Autodesk Inventor part; units mm, degrees
(part 2 of 3)
  line L955 (9.481, 12.2224) -> (9.3887, 12.173)
  line L956 (9.3887, 12.173) -> (9.2008, 12.0779)
  line L957 (9.2008, 12.0779) -> (8.8135, 11.9014)
  line L958 (8.8135, 11.9014) -> (8.4127, 11.7415)
  line L959 (8.4127, 11.7415) -> (7.9999, 11.5967)
  line L960 (7.9999, 11.5967) -> (7.5762, 11.4663)
  line L961 (7.5762, 11.4663) -> (7.1423, 11.3497)
  line L962 (7.1423, 11.3497) -> (6.777, 11.8009)
  line L963 (6.777, 11.8009) -> (6.9813, 12.201)
  line L964 (6.9813, 12.201) -> (7.1969, 12.5884)
  line L965 (7.1969, 12.5884) -> (7.4243, 12.9621)
  line L966 (7.4243, 12.9621) -> (7.6641, 13.3208)
  line L967 (7.6641, 13.3208) -> (7.9172, 13.663)
  line L968 (7.9172, 13.663) -> (8.0493, 13.827)
  line L969 (8.0493, 13.827) -> (8.1169, 13.907)
  line L970 (8.1169, 13.907) -> (8.1855, 13.9856)
  line L971 (8.1855, 13.9856) -> (7.7098, 14.6404)
  line L972 (7.7098, 14.6404) -> (7.6138, 14.5994)
  line L973 (7.6138, 14.5994) -> (7.5168, 14.5599)
  line L974 (7.5168, 14.5599) -> (7.32, 14.4849)
  line L975 (7.32, 14.4849) -> (6.9164, 14.3499)
  line L976 (6.9164, 14.3499) -> (6.5011, 14.2327)
  line L977 (6.5011, 14.2327) -> (6.0755, 14.1319)
  line L978 (6.0755, 14.1319) -> (5.6404, 14.0465)
  line L979 (5.6404, 14.0465) -> (5.1967, 13.9759)
  line L980 (5.1967, 13.9759) -> (4.8805, 14.4628)
  line L981 (4.8805, 14.4628) -> (5.1255, 14.8394)
  line L982 (5.1255, 14.8394) -> (5.3805, 15.2021)
  line L983 (5.3805, 15.2021) -> (5.6457, 15.55)
  line L984 (5.6457, 15.55) -> (5.9217, 15.8817)
  line L985 (5.9217, 15.8817) -> (6.2092, 16.1955)
  line L986 (6.2092, 16.1955) -> (6.3577, 16.3448)
  line L987 (6.3577, 16.3448) -> (6.4333, 16.4173)
  line L988 (6.4333, 16.4173) -> (6.5097, 16.4883)
  line L989 (6.5097, 16.4883) -> (6.1051, 17.1892)
  line L990 (6.1051, 17.1892) -> (6.0053, 17.1585)
  line L991 (6.0053, 17.1585) -> (5.9047, 17.1293)
  line L992 (5.9047, 17.1293) -> (5.7012, 17.0754)
  line L993 (5.7012, 17.0754) -> (5.2857, 16.9833)
  line L994 (5.2857, 16.9833) -> (4.8604, 16.9101)
  line L995 (4.8604, 16.9101) -> (4.4265, 16.8544)
  line L996 (4.4265, 16.8544) -> (3.9849, 16.8149)
  line L997 (3.9849, 16.8149) -> (3.5363, 16.7911)
  line L998 (3.5363, 16.7911) -> (3.2727, 17.3084)
  line L999 (3.2727, 17.3084) -> (3.5558, 17.6573)
  line L1000 (3.5558, 17.6573) -> (3.8472, 17.9913)
  line L1001 (3.8472, 17.9913) -> (4.1474, 18.3096)
  line L1002 (4.1474, 18.3096) -> (4.4565, 18.6106)
  line L1003 (4.4565, 18.6106) -> (4.7752, 18.8927)
  line L1004 (4.7752, 18.8927) -> (4.9385, 19.0256)
  line L1005 (4.9385, 19.0256) -> (5.0212, 19.0899)
  line L1006 (5.0212, 19.0899) -> (5.1047, 19.1525)
  line L1007 (5.1047, 19.1525) -> (4.7756, 19.8919)
  line L1008 (4.7756, 19.8919) -> (4.6731, 19.8717)
  line L1009 (4.6731, 19.8717) -> (4.5701, 19.8532)
  line L1010 (4.5701, 19.8532) -> (4.362, 19.8208)
  line L1011 (4.362, 19.8208) -> (3.9391, 19.7727)
  line L1012 (3.9391, 19.7727) -> (3.5085, 19.7444)
  line L1013 (3.5085, 19.7444) -> (3.0712, 19.7343)
  line L1014 (3.0712, 19.7343) -> (2.6279, 19.7412)
  line L1015 (2.6279, 19.7412) -> (2.1792, 19.7644)
  line L1016 (2.1792, 19.7644) -> (1.9712, 20.3064)
  line L1017 (1.9712, 20.3064) -> (2.2891, 20.6238)
  line L1018 (2.2891, 20.6238) -> (2.6139, 20.9256)
  line L1019 (2.6139, 20.9256) -> (2.9457, 21.2107)
  line L1020 (2.9457, 21.2107) -> (3.2846, 21.4778)
  line L1021 (3.2846, 21.4778) -> (3.631, 21.725)
  line L1022 (3.631, 21.725) -> (3.8074, 21.8401)
  line L1023 (3.8074, 21.8401) -> (3.8963, 21.8954)
  line L1024 (3.8963, 21.8954) -> (3.9859, 21.949)
  line L1025 (3.9859, 21.949) -> (3.7358, 22.7186)
  line L1026 (3.7358, 22.7186) -> (3.6319, 22.7093)
  line L1027 (3.6319, 22.7093) -> (3.5274, 22.7017)
  line L1028 (3.5274, 22.7017) -> (3.3171, 22.6913)
  line L1029 (3.3171, 22.6913) -> (2.8915, 22.6876)
  line L1030 (2.8915, 22.6876) -> (2.4603, 22.7045)
  line L1031 (2.4603, 22.7045) -> (2.0243, 22.7401)
  line L1032 (2.0243, 22.7401) -> (1.5842, 22.7933)
  line L1033 (1.5842, 22.7933) -> (1.1404, 22.8633)
  line L1034 (1.1404, 22.8633) -> (0.9901, 23.4241)
  line L1035 (0.9901, 23.4241) -> (1.3395, 23.7065)
  line L1036 (1.3395, 23.7065) -> (1.6941, 23.9727)
  line L1037 (1.6941, 23.9727) -> (2.0538, 24.2216)
  line L1038 (2.0538, 24.2216) -> (2.4188, 24.4518)
  line L1039 (2.4188, 24.4518) -> (2.7892, 24.6613)
  line L1040 (2.7892, 24.6613) -> (2.9766, 24.7575)
  line L1041 (2.9766, 24.7575) -> (3.0708, 24.8031)
  line L1042 (3.0708, 24.8031) -> (3.1655, 24.847)
  line L1043 (3.1655, 24.847) -> (2.9973, 25.6386)
  line L1044 (2.9973, 25.6386) -> (2.8929, 25.6402)
  line L1045 (2.8929, 25.6402) -> (2.7882, 25.6436)
  line L1046 (2.7882, 25.6436) -> (2.5779, 25.6552)
  line L1047 (2.5779, 25.6552) -> (2.1543, 25.696)
  line L1048 (2.1543, 25.696) -> (1.7273, 25.7578)
  line L1049 (1.7273, 25.7578) -> (1.2974, 25.8389)
  line L1050 (1.2974, 25.8389) -> (0.8652, 25.9378)
  line L1051 (0.8652, 25.9378) -> (0.4312, 26.0538)
  line L1052 (0.4312, 26.0538) -> (0.3404, 26.6272)
  line L1053 (0.3404, 26.6272) -> (0.7173, 26.8716)
  line L1054 (0.7173, 26.8716) -> (1.0978, 27.0992)
  line L1055 (1.0978, 27.0992) -> (1.4816, 27.3091)
  line L1056 (1.4816, 27.3091) -> (1.8686, 27.4999)
  line L1057 (1.8686, 27.4999) -> (2.2589, 27.6697)
  line L1058 (2.2589, 27.6697) -> (2.4553, 27.7456)
  line L1059 (2.4553, 27.7456) -> (2.5538, 27.7812)
  line L1060 (2.5538, 27.7812) -> (2.6526, 27.8149)
  line L1061 (2.6526, 27.8149) -> (2.568, 28.6198)
  line L1062 (2.568, 28.6198) -> (2.4644, 28.6323)
  line L1063 (2.4644, 28.6323) -> (2.3606, 28.6466)
  line L1064 (2.3606, 28.6466) -> (2.1527, 28.6801)
  line L1065 (2.1527, 28.6801) -> (1.7356, 28.765)
  line L1066 (1.7356, 28.765) -> (1.3174, 28.8711)
  line L1067 (1.3174, 28.8711) -> (0.8983, 28.9967)
  line L1068 (0.8983, 28.9967) -> (0.4789, 29.1403)
  line L1069 (0.4789, 29.1403) -> (0.0593, 29.3009)
  line L1070 (0.0593, 29.3009) -> (0.029, 29.8807)
  line L1071 (0.029, 29.8807) -> (0.4294, 30.0843)
  line L1072 (0.4294, 30.0843) -> (0.8316, 30.2709)
  line L1073 (0.8316, 30.2709) -> (1.2352, 30.4396)
  line L1074 (1.2352, 30.4396) -> (1.64, 30.5889)
  line L1075 (1.64, 30.5889) -> (2.0459, 30.7169)
  line L1076 (2.0459, 30.7169) -> (2.2492, 30.772)
  line L1077 (2.2492, 30.772) -> (2.3509, 30.797)
  line L1078 (2.3509, 30.797) -> (2.4527, 30.8203)
  line L1079 (2.4527, 30.8203) -> (2.4527, 31.6296)
  circle A0 centre (31.2249, 31.2249) radius 0.5
  line L1080 (62.4057, 32.859) -> (0.0441, 29.5908) construction
derived "Base_part.ipt"
sketch "Sketch7" plane through (0, 0, 0) normal (0, 1, 0) x (-1, 0, 0)
  line L0 (0.8173, 31.2129) -> (-0.8173, -31.2129) construction
  arc A0 (27.3185, 5) -> (4, 27.4827) centre (0, 0) ccw
  line L1 (5, 14.1421) -> (5, 27.3185)
  line L2 (4, 14.4568) -> (4, 27.4827)
  arc A1 (5, 27.3185) -> (4, 27.4827) centre (0, 0) ccw
  arc A2 (0.727, 27.7627) -> (27.4827, 4) centre (0, 0) ccw
  arc A3 (14.9718, 8.0526) -> (8.0526, 14.9718) centre (0, 0) ccw
  line L3 (16.7332, 7) -> (22.0027, 7)
  line L4 (7, 16.7332) -> (7, 22.0027)
  arc A4 (23.8539, 9.7572) -> (9.7572, 23.8539) centre (0, 0) ccw
  arc A5 (22.0027, 7) -> (23.8539, 9.7572) centre (22.0027, 9) ccw
  arc A6 (14.9718, 8.0526) -> (16.7332, 7) centre (16.7332, 9) ccw
  arc A7 (7, 16.7332) -> (8.0526, 14.9718) centre (9, 16.7332) ccw
  arc A8 (9.7572, 23.8539) -> (7, 22.0027) centre (9, 22.0027) ccw
  line L5 (0, 0) -> (0, -11.3594) construction
  arc A9 (14.1421, 5) -> (5, 14.1421) centre (0, 0) ccw
  line L6 (14.1421, 5) -> (27.3185, 5)
  line L7 (0, 0) -> (-23.3168, 0) construction
  line L8 (27.4827, 4) -> (14.4568, 4)
  arc A10 (14.4568, 4) -> (14.1421, 5) centre (0, 0) ccw
  arc A11 (4, 14.4568) -> (14.4568, 4) centre (0, 0) ccw
  arc A12 (5, 14.1421) -> (4, 14.4568) centre (0, 0) ccw
  arc A13 (27.3185, 5) -> (5, 27.3185) centre (0, 0) ccw
  arc A14 (27.4827, 4) -> (27.3185, 5) centre (0, 0) ccw
  arc A15 (4, 27.4827) -> (-14.6783, 23.5764) centre (0, 0) ccw
  arc A16 (-4, 14.4568) -> (-5, 14.1421) centre (0, 0) ccw
  line L9 (-4, 27.4827) -> (-4, 14.4568)
  arc A17 (-4, 27.4827) -> (-5, 27.3185) centre (0, 0) ccw
  line L10 (-5, 14.1421) -> (-5, 27.3185)
  arc A18 (-14.1421, 5) -> (-14.4568, 4) centre (0, 0) ccw
  line L11 (-14.1421, 5) -> (-27.3184, 5)
  line L12 (-14.4568, 4) -> (-27.4827, 4)
  arc A19 (-27.3184, 5) -> (-27.4827, 4) centre (0, 0) ccw
  arc A20 (-23.8538, 9.7572) -> (-22.0027, 7) centre (-22.0027, 9) ccw
  arc A21 (-9.7572, 23.8539) -> (-23.8538, 9.7572) centre (0, 0) ccw
  arc A22 (-8.0526, 14.9718) -> (-14.9718, 8.0526) centre (0, 0) ccw
  arc A23 (-16.7332, 7) -> (-14.9718, 8.0526) centre (-16.7332, 9) ccw
  line L13 (-16.7332, 7) -> (-22.0027, 7)
  arc A24 (-8.0526, 14.9718) -> (-7, 16.7332) centre (-9, 16.7332) ccw
  arc A25 (-7, 22.0027) -> (-9.7572, 23.8539) centre (-9, 22.0027) ccw
  line L14 (-7, 16.7332) -> (-7, 22.0027)
  arc A26 (-14.4568, -4) -> (-14.1421, -5) centre (0, 0) ccw
  line L15 (-27.4827, -4) -> (-14.4568, -4)
  arc A27 (-27.4827, -4) -> (-27.3184, -5) centre (0, 0) ccw
  line L16 (-14.1421, -5) -> (-27.3184, -5)
  arc A28 (-5, -14.1421) -> (-4, -14.4568) centre (0, 0) ccw
  line L17 (-5, -14.1421) -> (-5, -27.3184)
  line L18 (-4, -14.4568) -> (-4, -27.4827)
  arc A29 (-5, -27.3184) -> (-4, -27.4827) centre (0, 0) ccw
  arc A30 (-9.7572, -23.8538) -> (-7, -22.0027) centre (-9, -22.0027) ccw
  arc A31 (-23.8538, -9.7572) -> (-9.7572, -23.8538) centre (0, 0) ccw
  arc A32 (-14.9718, -8.0526) -> (-8.0526, -14.9718) centre (0, 0) ccw
  arc A33 (-7, -16.7332) -> (-8.0526, -14.9718) centre (-9, -16.7332) ccw
  line L19 (-7, -16.7332) -> (-7, -22.0027)
  arc A34 (-14.9718, -8.0526) -> (-16.7332, -7) centre (-16.7332, -9) ccw
  arc A35 (-22.0027, -7) -> (-23.8538, -9.7572) centre (-22.0027, -9) ccw
  line L20 (-16.7332, -7) -> (-22.0027, -7)
  arc A36 (4, -14.4568) -> (5, -14.1421) centre (0, 0) ccw
  line L21 (4, -27.4827) -> (4, -14.4568)
  arc A37 (4, -27.4827) -> (5, -27.3184) centre (0, 0) ccw
  line L22 (5, -14.1421) -> (5, -27.3184)
  arc A38 (14.1421, -5) -> (14.4568, -4) centre (0, 0) ccw
  line L23 (14.1421, -5) -> (27.3185, -5)
  line L24 (14.4568, -4) -> (27.4827, -4)
  arc A39 (27.3185, -5) -> (27.4827, -4) centre (0, 0) ccw
  arc A40 (23.8539, -9.7572) -> (22.0027, -7) centre (22.0027, -9) ccw
  arc A41 (9.7572, -23.8538) -> (23.8539, -9.7572) centre (0, 0) ccw
  arc A42 (8.0526, -14.9718) -> (14.9718, -8.0526) centre (0, 0) ccw
  arc A43 (16.7332, -7) -> (14.9718, -8.0526) centre (16.7332, -9) ccw
  line L25 (16.7332, -7) -> (22.0027, -7)
  arc A44 (8.0526, -14.9718) -> (7, -16.7332) centre (9, -16.7332) ccw
  arc A45 (7, -22.0027) -> (9.7572, -23.8538) centre (9, -22.0027) ccw
  line L26 (7, -16.7332) -> (7, -22.0027)
  line L27 (-28.6518, 2.6609) -> (-28.7514, 2.692)
  line L28 (-28.7514, 2.692) -> (-28.8508, 2.725)
  line L29 (-28.8508, 2.725) -> (-29.0492, 2.7958)
  line L30 (-29.0492, 2.7958) -> (-29.4438, 2.9552)
  line L31 (-29.4438, 2.9552) -> (-29.8357, 3.1359)
  line L32 (-29.8357, 3.1359) -> (-30.2248, 3.3356)
  line L33 (-30.2248, 3.3356) -> (-30.6111, 3.5533)
  line L34 (-30.6111, 3.5533) -> (-30.9943, 3.7877)
  line L35 (-30.9943, 3.7877) -> (-30.9185, 4.3633)
  line L36 (-30.9185, 4.3633) -> (-30.4877, 4.4905)
  line L37 (-30.4877, 4.4905) -> (-30.0582, 4.6008)
  line L38 (-30.0582, 4.6008) -> (-29.6306, 4.693)
  line L39 (-29.6306, 4.693) -> (-29.2054, 4.7661)
  line L40 (-29.2054, 4.7661) -> (-28.7829, 4.8179)
  line L41 (-28.7829, 4.8179) -> (-28.573, 4.835)
  line L42 (-28.573, 4.835) -> (-28.4685, 4.8411)
  line L43 (-28.4685, 4.8411) -> (-28.3642, 4.8454)
  line L44 (-28.3642, 4.8454) -> (-28.2167, 5.6412)
  line L45 (-28.2167, 5.6412) -> (-28.3125, 5.6826)
  line L46 (-28.3125, 5.6826) -> (-28.408, 5.7258)
  line L47 (-28.408, 5.7258) -> (-28.5978, 5.817)
  line L48 (-28.5978, 5.817) -> (-28.9736, 6.0168)
  line L49 (-28.9736, 6.0168) -> (-29.3444, 6.2373)
  line L50 (-29.3444, 6.2373) -> (-29.7105, 6.4767)
  line L51 (-29.7105, 6.4767) -> (-30.072, 6.7335)
  line L52 (-30.072, 6.7335) -> (-30.4286, 7.0067)
  line L53 (-30.4286, 7.0067) -> (-30.2931, 7.5713)
  line L54 (-30.2931, 7.5713) -> (-29.8513, 7.6528)
  line L55 (-29.8513, 7.6528) -> (-29.4127, 7.7175)
  line L56 (-29.4127, 7.7175) -> (-28.9778, 7.7646)
  line L57 (-28.9778, 7.7646) -> (-28.5472, 7.7928)
  line L58 (-28.5472, 7.7928) -> (-28.1217, 7.8002)
  line L59 (-28.1217, 7.8002) -> (-27.9111, 7.7952)
  line L60 (-27.9111, 7.7952) -> (-27.8065, 7.7904)
  line L61 (-27.8065, 7.7904) -> (-27.7023, 7.7838)
  line L62 (-27.7023, 7.7838) -> (-27.4725, 8.5597)
  line L63 (-27.4725, 8.5597) -> (-27.5634, 8.6109)
  line L64 (-27.5634, 8.6109) -> (-27.6538, 8.6638)
  line L65 (-27.6538, 8.6638) -> (-27.8331, 8.7744)
  line L66 (-27.8331, 8.7744) -> (-28.1859, 9.0124)
  line L67 (-28.1859, 9.0124) -> (-28.5317, 9.2705)
  line L68 (-28.5317, 9.2705) -> (-28.8708, 9.5468)
  line L69 (-28.8708, 9.5468) -> (-29.2034, 9.84)
  line L70 (-29.2034, 9.84) -> (-29.5295, 10.149)
  line L71 (-29.5295, 10.149) -> (-29.3357, 10.6963)
  line L72 (-29.3357, 10.6963) -> (-28.8878, 10.7312)
  line L73 (-28.8878, 10.7312) -> (-28.4448, 10.7497)
  line L74 (-28.4448, 10.7497) -> (-28.0074, 10.751)
  line L75 (-28.0074, 10.751) -> (-27.5762, 10.734)
  line L76 (-27.5762, 10.734) -> (-27.1523, 10.697)
  line L77 (-27.1523, 10.697) -> (-26.9434, 10.67)
  line L78 (-26.9434, 10.67) -> (-26.8399, 10.6543)
  line L79 (-26.8399, 10.6543) -> (-26.7369, 10.6368)
  line L80 (-26.7369, 10.6368) -> (-26.4272, 11.3845)
  line L81 (-26.4272, 11.3845) -> (-26.5123, 11.4449)
  line L82 (-26.5123, 11.4449) -> (-26.5967, 11.507)
  line L83 (-26.5967, 11.507) -> (-26.7634, 11.6356)
  line L84 (-26.7634, 11.6356) -> (-27.0895, 11.9092)
  line L85 (-27.0895, 11.9092) -> (-27.4064, 12.2021)
  line L86 (-27.4064, 12.2021) -> (-27.7147, 12.5124)
  line L87 (-27.7147, 12.5124) -> (-28.0148, 12.8387)
  line L88 (-28.0148, 12.8387) -> (-28.3069, 13.1801)
  line L89 (-28.3069, 13.1801) -> (-28.0569, 13.7041)
  line L90 (-28.0569, 13.7041) -> (-27.6078, 13.692)
  line L91 (-27.6078, 13.692) -> (-27.1654, 13.6641)
  line L92 (-27.1654, 13.6641) -> (-26.7302, 13.6197)
  line L93 (-26.7302, 13.6197) -> (-26.3032, 13.5577)
  line L94 (-26.3032, 13.5577) -> (-25.8854, 13.4766)
  line L95 (-25.8854, 13.4766) -> (-25.6805, 13.4279)
  line L96 (-25.6805, 13.4279) -> (-25.5791, 13.4014)
  line L97 (-25.5791, 13.4014) -> (-25.4786, 13.3733)
  line L98 (-25.4786, 13.3733) -> (-25.0925, 14.0845)
  line L99 (-25.0925, 14.0845) -> (-25.1708, 14.1535)
  line L100 (-25.1708, 14.1535) -> (-25.2482, 14.2241)
  line L101 (-25.2482, 14.2241) -> (-25.4006, 14.3695)
  line L102 (-25.4006, 14.3695) -> (-25.6962, 14.6756)
  line L103 (-25.6962, 14.6756) -> (-25.9808, 15)
  line L104 (-25.9808, 15) -> (-26.255, 15.3408)
  line L105 (-26.255, 15.3408) -> (-26.5194, 15.6967)
  line L106 (-26.5194, 15.6967) -> (-26.7741, 16.0667)
  line L107 (-26.7741, 16.0667) -> (-26.4708, 16.5618)
  line L108 (-26.4708, 16.5618) -> (-26.0254, 16.5028)
  line L109 (-26.0254, 16.5028) -> (-25.5883, 16.4288)
  line L110 (-25.5883, 16.4288) -> (-25.1601, 16.3392)
  line L111 (-25.1601, 16.3392) -> (-24.7419, 16.2329)
  line L112 (-24.7419, 16.2329) -> (-24.3349, 16.1085)
  line L113 (-24.3349, 16.1085) -> (-24.1362, 16.0387)
  line L114 (-24.1362, 16.0387) -> (-24.0382, 16.0018)
  line L115 (-24.0382, 16.0018) -> (-23.9412, 15.9633)
  line L116 (-23.9412, 15.9633) -> (-23.4828, 16.6303)
  line L117 (-23.4828, 16.6303) -> (-23.5534, 16.7071)
  line L118 (-23.5534, 16.7071) -> (-23.6231, 16.7853)
  line L119 (-23.6231, 16.7853) -> (-23.7594, 16.9458)
  line L120 (-23.7594, 16.9458) -> (-24.0214, 17.2812)
  line L121 (-24.0214, 17.2812) -> (-24.2705, 17.6336)
  line L122 (-24.2705, 17.6336) -> (-24.5076, 18.0012)
  line L123 (-24.5076, 18.0012) -> (-24.7333, 18.3827)
  line L124 (-24.7333, 18.3827) -> (-24.948, 18.7774)
  line L125 (-24.948, 18.7774) -> (-24.5946, 19.238)
  line L126 (-24.5946, 19.238) -> (-24.1578, 19.1328)
  line L127 (-24.1578, 19.1328) -> (-23.7308, 19.0135)
  line L128 (-23.7308, 19.0135) -> (-23.3144, 18.8796)
  line L129 (-23.3144, 18.8796) -> (-22.9096, 18.7302)
  line L130 (-22.9096, 18.7302) -> (-22.5178, 18.5639)
  line L131 (-22.5178, 18.5639) -> (-22.3275, 18.4738)
  line L132 (-22.3275, 18.4738) -> (-22.2339, 18.4268)
  line L133 (-22.2339, 18.4268) -> (-22.1414, 18.3784)
  line L134 (-22.1414, 18.3784) -> (-21.6158, 18.9938)
  line L135 (-21.6158, 18.9938) -> (-21.6781, 19.0776)
  line L136 (-21.6781, 19.0776) -> (-21.7391, 19.1626)
  line L137 (-21.7391, 19.1626) -> (-21.8579, 19.3365)
  line L138 (-21.8579, 19.3365) -> (-22.0835, 19.6974)
  line L139 (-22.0835, 19.6974) -> (-22.2943, 20.0739)
  line L140 (-22.2943, 20.0739) -> (-22.4917, 20.4643)
  line L141 (-22.4917, 20.4643) -> (-22.6763, 20.8674)
  line L142 (-22.6763, 20.8674) -> (-22.8486, 21.2823)
  line L143 (-22.8486, 21.2823) -> (-22.4489, 21.7035)
  line L144 (-22.4489, 21.7035) -> (-22.0256, 21.5531)
  line L145 (-22.0256, 21.5531) -> (-21.6134, 21.3899)
  line L146 (-21.6134, 21.3899) -> (-21.2132, 21.2132)
  line L147 (-21.2132, 21.2132) -> (-20.8262, 21.0223)
  line L148 (-20.8262, 21.0223) -> (-20.454, 20.816)
  line L149 (-20.454, 20.816) -> (-20.2741, 20.7064)
  line L150 (-20.2741, 20.7064) -> (-20.1859, 20.6499)
  line L151 (-20.1859, 20.6499) -> (-20.099, 20.5921)
  line L152 (-20.099, 20.5921) -> (-19.512, 21.1492)
  line L153 (-19.512, 21.1492) -> (-19.5652, 21.239)
  line L154 (-19.5652, 21.239) -> (-19.617, 21.33)
  line L155 (-19.617, 21.33) -> (-19.717, 21.5154)
  line L156 (-19.717, 21.5154) -> (-19.9035, 21.8979)
  line L157 (-19.9035, 21.8979) -> (-20.0739, 22.2943)
  line L158 (-20.0739, 22.2943) -> (-20.2294, 22.7032)
  line L159 (-20.2294, 22.7032) -> (-20.3709, 23.1234)
  line L160 (-20.3709, 23.1234) -> (-20.4988, 23.5541)
  line L161 (-20.4988, 23.5541) -> (-20.0573, 23.9311)
  line L162 (-20.0573, 23.9311) -> (-19.652, 23.7374)
  line L163 (-19.652, 23.7374) -> (-19.2591, 23.5319)
  line L164 (-19.2591, 23.5319) -> (-18.8796, 23.3144)
  line L165 (-18.8796, 23.3144) -> (-18.5147, 23.0841)
  line L166 (-18.5147, 23.0841) -> (-18.1661, 22.84)
  line L167 (-18.1661, 22.84) -> (-17.9987, 22.7122)
  line L168 (-17.9987, 22.7122) -> (-17.9169, 22.6468)
  line L169 (-17.9169, 22.6468) -> (-17.8365, 22.5802)
  line L170 (-17.8365, 22.5802) -> (-17.1944, 23.0729)
  line L171 (-17.1944, 23.0729) -> (-17.2379, 23.1678)
  line L172 (-17.2379, 23.1678) -> (-17.2799, 23.2637)
  line L173 (-17.2799, 23.2637) -> (-17.36, 23.4585)
  line L174 (-17.36, 23.4585) -> (-17.5056, 23.8584)
  line L175 (-17.5056, 23.8584) -> (-17.6336, 24.2705)
  line L176 (-17.6336, 24.2705) -> (-17.7455, 24.6934)
  line L177 (-17.7455, 24.6934) -> (-17.8422, 25.1261)
  line L178 (-17.8422, 25.1261) -> (-17.9245, 25.5677)
  line L179 (-17.9245, 25.5677) -> (-17.446, 25.8966)
  line L180 (-17.446, 25.8966) -> (-17.0631, 25.6615)
  line L181 (-17.0631, 25.6615) -> (-16.6939, 25.4161)
  line L182 (-16.6939, 25.4161) -> (-16.3392, 25.1601)
  line L183 (-16.3392, 25.1601) -> (-16.0003, 24.8929)
  line L184 (-16.0003, 24.8929) -> (-15.6791, 24.6137)
  line L185 (-15.6791, 24.6137) -> (-15.526, 24.4692)
  line L186 (-15.526, 24.4692) -> (-15.4515, 24.3955)
  line L187 (-15.4515, 24.3955) -> (-15.3785, 24.3209)
  line L188 (-15.3785, 24.3209) -> (-14.6884, 24.7438)
  line L189 (-14.6884, 24.7438) -> (-14.7218, 24.8427)
  line L190 (-14.7218, 24.8427) -> (-14.7535, 24.9425)
  line L191 (-14.7535, 24.9425) -> (-14.8128, 25.1446)
  line L192 (-14.8128, 25.1446) -> (-14.9158, 25.5575)
  line L193 (-14.9158, 25.5575) -> (-15, 25.9808)
  line L194 (-15, 25.9808) -> (-15.0671, 26.413)
  line L195 (-15.0671, 26.413) -> (-15.1181, 26.8534)
  line L196 (-15.1181, 26.8534) -> (-15.1537, 27.3013)
  line L197 (-15.1537, 27.3013) -> (-14.6435, 27.5783)
  line L198 (-14.6435, 27.5783) -> (-14.2873, 27.3045)
  line L199 (-14.2873, 27.3045) -> (-13.9457, 27.0219)
  line L200 (-13.9457, 27.0219) -> (-13.6197, 26.7302)
  line L201 (-13.6197, 26.7302) -> (-13.3106, 26.4291)
  line L202 (-13.3106, 26.4291) -> (-13.0204, 26.1178)
  line L203 (-13.0204, 26.1178) -> (-12.8832, 25.958)
  line L204 (-12.8832, 25.958) -> (-12.8168, 25.877)
  line L205 (-12.8168, 25.877) -> (-12.752, 25.7952)
  line L206 (-12.752, 25.7952) -> (-12.0215, 26.1436)
  line L207 (-12.0215, 26.1436) -> (-12.0444, 26.2455)
  line L208 (-12.0444, 26.2455) -> (-12.0655, 26.348)
  line L209 (-12.0655, 26.348) -> (-12.1033, 26.5552)
  line L210 (-12.1033, 26.5552) -> (-12.1626, 26.9767)
  line L211 (-12.1626, 26.9767) -> (-12.2021, 27.4064)
  line L212 (-12.2021, 27.4064) -> (-12.2236, 27.8433)
  line L213 (-12.2236, 27.8433) -> (-12.2283, 28.2866)
  line L214 (-12.2283, 28.2866) -> (-12.2169, 28.7357)
  line L215 (-12.2169, 28.7357) -> (-11.6805, 28.9579)
  line L216 (-11.6805, 28.9579) -> (-11.3549, 28.6484)
  line L217 (-11.3549, 28.6484) -> (-11.0447, 28.3316)
  line L218 (-11.0447, 28.3316) -> (-10.751, 28.0074)
  line L219 (-10.751, 28.0074) -> (-10.4751, 27.6756)
  line L220 (-10.4751, 27.6756) -> (-10.219, 27.3357)
  line L221 (-10.219, 27.3357) -> (-10.0993, 27.1625)
  line L222 (-10.0993, 27.1625) -> (-10.0417, 27.075)
  line L223 (-10.0417, 27.075) -> (-9.9858, 26.9868)
  line L224 (-9.9858, 26.9868) -> (-9.2229, 27.257)
  line L225 (-9.2229, 27.257) -> (-9.235, 27.3607)
  line L226 (-9.235, 27.3607) -> (-9.2453, 27.4649)
  line L227 (-9.2453, 27.4649) -> (-9.2613, 27.6749)
  line L228 (-9.2613, 27.6749) -> (-9.2761, 28.1002)
  line L229 (-9.2761, 28.1002) -> (-9.2705, 28.5317)
  line L230 (-9.2705, 28.5317) -> (-9.2463, 28.9685)
  line L231 (-9.2463, 28.9685) -> (-9.2046, 29.4098)
  line L232 (-9.2046, 29.4098) -> (-9.1463, 29.8553)
  line L233 (-9.1463, 29.8553) -> (-8.5896, 30.0202)
  line L234 (-8.5896, 30.0202) -> (-8.2981, 29.6783)
  line L235 (-8.2981, 29.6783) -> (-8.0228, 29.3309)
  line L236 (-8.0228, 29.3309) -> (-7.7646, 28.9778)
  line L237 (-7.7646, 28.9778) -> (-7.5249, 28.619)
  line L238 (-7.5249, 28.619) -> (-7.3057, 28.2542)
  line L239 (-7.3057, 28.2542) -> (-7.2047, 28.0694)
  line L240 (-7.2047, 28.0694) -> (-7.1566, 27.9763)
  line L241 (-7.1566, 27.9763) -> (-7.1102, 27.8828)
  line L242 (-7.1102, 27.8828) -> (-6.3233, 28.0717)
  line L243 (-6.3233, 28.0717) -> (-6.3244, 28.1761)
  line L244 (-6.3244, 28.1761) -> (-6.3238, 28.2808)
  line L245 (-6.3238, 28.2808) -> (-6.3177, 28.4913)
  line L246 (-6.3177, 28.4913) -> (-6.288, 28.9159)
  line L247 (-6.288, 28.9159) -> (-6.2373, 29.3444)
  line L248 (-6.2373, 29.3444) -> (-6.1676, 29.7763)
  line L249 (-6.1676, 29.7763) -> (-6.08, 30.2109)
  line L250 (-6.08, 30.2109) -> (-5.9755, 30.6478)
  line L251 (-5.9755, 30.6478) -> (-5.4046, 30.7536)
  line L252 (-5.4046, 30.7536) -> (-5.1504, 30.3832)
  line L253 (-5.1504, 30.3832) -> (-4.9129, 30.0088)
  line L254 (-4.9129, 30.0088) -> (-4.693, 29.6306)
  line L255 (-4.693, 29.6306) -> (-4.4922, 29.2487)
  line L256 (-4.4922, 29.2487) -> (-4.3123, 28.863)
  line L257 (-4.3123, 28.863) -> (-4.2312, 28.6687)
  line L258 (-4.2312, 28.6687) -> (-4.1931, 28.5711)
  line L259 (-4.1931, 28.5711) -> (-4.1567, 28.4733)
  line L260 (-4.1567, 28.4733) -> (-3.3543, 28.5789)
  line L261 (-3.3543, 28.5789) -> (-3.3446, 28.6828)
  line L262 (-3.3446, 28.6828) -> (-3.333, 28.7869)
  line L263 (-3.333, 28.7869) -> (-3.305, 28.9957)
  line L264 (-3.305, 28.9957) -> (-3.231, 29.4148)
  line L265 (-3.231, 29.4148) -> (-3.1359, 29.8357)
  line L266 (-3.1359, 29.8357) -> (-3.0213, 30.2578)
  line L267 (-3.0213, 30.2578) -> (-2.8888, 30.6809)
  line L268 (-2.8888, 30.6809) -> (-2.7392, 31.1045)
  line L269 (-2.7392, 31.1045) -> (-2.1604, 31.1501)
  line L270 (-2.1604, 31.1501) -> (-1.9463, 30.7551)
  line L271 (-1.9463, 30.7551) -> (-1.7492, 30.3579)
  line L272 (-1.7492, 30.3579) -> (-1.5701, 29.9589)
  line L273 (-1.5701, 29.9589) -> (-1.4102, 29.5581)
  line L274 (-1.4102, 29.5581) -> (-1.2716, 29.1557)
  line L275 (-1.2716, 29.1557) -> (-1.2113, 28.9539)
  line L276 (-1.2113, 28.9539) -> (-1.1836, 28.8529)
  line L277 (-1.1836, 28.8529) -> (-1.1577, 28.7518)
  line L278 (-1.1577, 28.7518) -> (-0.3487, 28.773)
  line L279 (-0.3487, 28.773) -> (-0.3281, 28.8753)
  line L280 (-0.3281, 28.8753) -> (-0.3057, 28.9776)
  line L281 (-0.3057, 28.9776) -> (-0.256, 29.1823)
  line L282 (-0.256, 29.1823) -> (-0.1387, 29.5914)
  line L283 (-0.1387, 29.5914) -> (0, 30)
  line L284 (0, 30) -> (0.158, 30.4079)
  line L285 (0.158, 30.4079) -> (0.3341, 30.8148)
  line L286 (0.3341, 30.8148) -> (0.5271, 31.2205)
  line L287 (0.5271, 31.2205) -> (1.1075, 31.2053)
  line L288 (1.1075, 31.2053) -> (1.2791, 30.79)
  line L289 (1.2791, 30.79) -> (1.4336, 30.3745)
  line L290 (1.4336, 30.3745) -> (1.5701, 29.9589)
  line L291 (1.5701, 29.9589) -> (1.6872, 29.5436)
  line L292 (1.6872, 29.5436) -> (1.7829, 29.1289)
  line L293 (1.7829, 29.1289) -> (1.8218, 28.9219)
  line L294 (1.8218, 28.9219) -> (1.8388, 28.8186)
  line L295 (1.8388, 28.8186) -> (1.854, 28.7153)
  line L296 (1.854, 28.7153) -> (2.6608, 28.6518)
  line L297 (2.6608, 28.6518) -> (2.692, 28.7514)
  line L298 (2.692, 28.7514) -> (2.725, 28.8508)
  line L299 (2.725, 28.8508) -> (2.7958, 29.0492)
  line L300 (2.7958, 29.0492) -> (2.9552, 29.4438)
  line L301 (2.9552, 29.4438) -> (3.1359, 29.8357)
  line L302 (3.1359, 29.8357) -> (3.3356, 30.2248)
  line L303 (3.3356, 30.2248) -> (3.5533, 30.6111)
  line L304 (3.5533, 30.6111) -> (3.7877, 30.9943)
  line L305 (3.7877, 30.9943) -> (4.3633, 30.9185)
  line L306 (4.3633, 30.9185) -> (4.4905, 30.4877)
  line L307 (4.4905, 30.4877) -> (4.6008, 30.0582)
  line L308 (4.6008, 30.0582) -> (4.693, 29.6307)
  line L309 (4.693, 29.6307) -> (4.7661, 29.2054)
  line L310 (4.7661, 29.2054) -> (4.8179, 28.7829)
  line L311 (4.8179, 28.7829) -> (4.835, 28.5731)
  line L312 (4.835, 28.5731) -> (4.8411, 28.4685)
  line L313 (4.8411, 28.4685) -> (4.8454, 28.3642)
  line L314 (4.8454, 28.3642) -> (5.6412, 28.2167)
  line L315 (5.6412, 28.2167) -> (5.6826, 28.3125)
  line L316 (5.6826, 28.3125) -> (5.7258, 28.408)
  line L317 (5.7258, 28.408) -> (5.817, 28.5978)
  line L318 (5.817, 28.5978) -> (6.0168, 28.9736)
  line L319 (6.0168, 28.9736) -> (6.2373, 29.3444)
  line L320 (6.2373, 29.3444) -> (6.4767, 29.7106)
  line L321 (6.4767, 29.7106) -> (6.7335, 30.072)
  line L322 (6.7335, 30.072) -> (7.0067, 30.4286)
  line L323 (7.0067, 30.4286) -> (7.5713, 30.2931)
  line L324 (7.5713, 30.2931) -> (7.6528, 29.8513)
  line L325 (7.6528, 29.8513) -> (7.7175, 29.4127)
  line L326 (7.7175, 29.4127) -> (7.7646, 28.9778)
  line L327 (7.7646, 28.9778) -> (7.7928, 28.5472)
  line L328 (7.7928, 28.5472) -> (7.8002, 28.1217)
  line L329 (7.8002, 28.1217) -> (7.7952, 27.9111)
  line L330 (7.7952, 27.9111) -> (7.7904, 27.8065)
  line L331 (7.7904, 27.8065) -> (7.7838, 27.7023)
  line L332 (7.7838, 27.7023) -> (8.5597, 27.4725)
  line L333 (8.5597, 27.4725) -> (8.6109, 27.5634)
  line L334 (8.6109, 27.5634) -> (8.6638, 27.6538)
  line L335 (8.6638, 27.6538) -> (8.7744, 27.8331)
  line L336 (8.7744, 27.8331) -> (9.0124, 28.1859)
  line L337 (9.0124, 28.1859) -> (9.2705, 28.5317)
  line L338 (9.2705, 28.5317) -> (9.5468, 28.8708)
  line L339 (9.5468, 28.8708) -> (9.84, 29.2034)
  line L340 (9.84, 29.2034) -> (10.149, 29.5295)
  line L341 (10.149, 29.5295) -> (10.6963, 29.3357)
  line L342 (10.6963, 29.3357) -> (10.7312, 28.8878)
  line L343 (10.7312, 28.8878) -> (10.7497, 28.4448)
  line L344 (10.7497, 28.4448) -> (10.751, 28.0074)
  line L345 (10.751, 28.0074) -> (10.734, 27.5762)
  line L346 (10.734, 27.5762) -> (10.697, 27.1523)
  line L347 (10.697, 27.1523) -> (10.67, 26.9434)
  line L348 (10.67, 26.9434) -> (10.6543, 26.8398)
  line L349 (10.6543, 26.8398) -> (10.6368, 26.7369)
  line L350 (10.6368, 26.7369) -> (11.3845, 26.4272)
  line L351 (11.3845, 26.4272) -> (11.4449, 26.5123)
  line L352 (11.4449, 26.5123) -> (11.507, 26.5967)
  line L353 (11.507, 26.5967) -> (11.6356, 26.7635)
  line L354 (11.6356, 26.7635) -> (11.9092, 27.0895)
  line L355 (11.9092, 27.0895) -> (12.2021, 27.4064)
  line L356 (12.2021, 27.4064) -> (12.5124, 27.7147)
  line L357 (12.5124, 27.7147) -> (12.8387, 28.0148)
  line L358 (12.8387, 28.0148) -> (13.1801, 28.3069)
  line L359 (13.1801, 28.3069) -> (13.7041, 28.057)
  line L360 (13.7041, 28.057) -> (13.692, 27.6078)
  line L361 (13.692, 27.6078) -> (13.6641, 27.1654)
  line L362 (13.6641, 27.1654) -> (13.6197, 26.7302)
  line L363 (13.6197, 26.7302) -> (13.5577, 26.3032)
  line L364 (13.5577, 26.3032) -> (13.4766, 25.8854)
  line L365 (13.4766, 25.8854) -> (13.4279, 25.6805)
  line L366 (13.4279, 25.6805) -> (13.4014, 25.5791)
  line L367 (13.4014, 25.5791) -> (13.3733, 25.4786)
  line L368 (13.3733, 25.4786) -> (14.0845, 25.0925)
  line L369 (14.0845, 25.0925) -> (14.1535, 25.1708)
  line L370 (14.1535, 25.1708) -> (14.2241, 25.2482)
  line L371 (14.2241, 25.2482) -> (14.3695, 25.4006)
  line L372 (14.3695, 25.4006) -> (14.6756, 25.6962)
  line L373 (14.6756, 25.6962) -> (15, 25.9808)
  line L374 (15, 25.9808) -> (15.3408, 26.255)
  line L375 (15.3408, 26.255) -> (15.6967, 26.5194)
  line L376 (15.6967, 26.5194) -> (16.0667, 26.7741)
  line L377 (16.0667, 26.7741) -> (16.5618, 26.4708)
  line L378 (16.5618, 26.4708) -> (16.5028, 26.0254)
  line L379 (16.5028, 26.0254) -> (16.4288, 25.5883)
  line L380 (16.4288, 25.5883) -> (16.3392, 25.1601)
  line L381 (16.3392, 25.1601) -> (16.2329, 24.7419)
  line L382 (16.2329, 24.7419) -> (16.1085, 24.3349)
  line L383 (16.1085, 24.3349) -> (16.0387, 24.1362)
  line L384 (16.0387, 24.1362) -> (16.0018, 24.0382)
  line L385 (16.0018, 24.0382) -> (15.9633, 23.9412)
  line L386 (15.9633, 23.9412) -> (16.6303, 23.4828)
  line L387 (16.6303, 23.4828) -> (16.7071, 23.5534)
  line L388 (16.7071, 23.5534) -> (16.7853, 23.6231)
  line L389 (16.7853, 23.6231) -> (16.9458, 23.7594)
  line L390 (16.9458, 23.7594) -> (17.2812, 24.0214)
  line L391 (17.2812, 24.0214) -> (17.6336, 24.2705)
  line L392 (17.6336, 24.2705) -> (18.0012, 24.5076)
  line L393 (18.0012, 24.5076) -> (18.3827, 24.7333)
  line L394 (18.3827, 24.7333) -> (18.7774, 24.948)
  line L395 (18.7774, 24.948) -> (19.238, 24.5946)
  line L396 (19.238, 24.5946) -> (19.1328, 24.1578)
  line L397 (19.1328, 24.1578) -> (19.0135, 23.7308)
  line L398 (19.0135, 23.7308) -> (18.8796, 23.3144)
  line L399 (18.8796, 23.3144) -> (18.7302, 22.9095)
  line L400 (18.7302, 22.9095) -> (18.5639, 22.5178)
  line L401 (18.5639, 22.5178) -> (18.4738, 22.3275)
  line L402 (18.4738, 22.3275) -> (18.4268, 22.2339)
  line L403 (18.4268, 22.2339) -> (18.3784, 22.1414)
  line L404 (18.3784, 22.1414) -> (18.9938, 21.6158)
  line L405 (18.9938, 21.6158) -> (19.0776, 21.6781)
  line L406 (19.0776, 21.6781) -> (19.1626, 21.7391)
  line L407 (19.1626, 21.7391) -> (19.3365, 21.8579)
  line L408 (19.3365, 21.8579) -> (19.6974, 22.0835)
  line L409 (19.6974, 22.0835) -> (20.0739, 22.2943)
  line L410 (20.0739, 22.2943) -> (20.4643, 22.4917)
  line L411 (20.4643, 22.4917) -> (20.8674, 22.6763)
  line L412 (20.8674, 22.6763) -> (21.2823, 22.8486)
  line L413 (21.2823, 22.8486) -> (21.7035, 22.4489)
  line L414 (21.7035, 22.4489) -> (21.5531, 22.0256)
  line L415 (21.5531, 22.0256) -> (21.3899, 21.6134)
  line L416 (21.3899, 21.6134) -> (21.2132, 21.2132)
  line L417 (21.2132, 21.2132) -> (21.0223, 20.8262)
  line L418 (21.0223, 20.8262) -> (20.816, 20.454)
  line L419 (20.816, 20.454) -> (20.7064, 20.2741)
  line L420 (20.7064, 20.2741) -> (20.6499, 20.1859)
  line L421 (20.6499, 20.1859) -> (20.5921, 20.099)
  line L422 (20.5921, 20.099) -> (21.1492, 19.512)
  line L423 (21.1492, 19.512) -> (21.239, 19.5652)
  line L424 (21.239, 19.5652) -> (21.33, 19.617)
  line L425 (21.33, 19.617) -> (21.5154, 19.717)
  line L426 (21.5154, 19.717) -> (21.8979, 19.9035)
  line L427 (21.8979, 19.9035) -> (22.2943, 20.0739)
  line L428 (22.2943, 20.0739) -> (22.7032, 20.2294)
  line L429 (22.7032, 20.2294) -> (23.1234, 20.3709)
  line L430 (23.1234, 20.3709) -> (23.5541, 20.4988)
  line L431 (23.5541, 20.4988) -> (23.9311, 20.0573)
  line L432 (23.9311, 20.0573) -> (23.7374, 19.652)
  line L433 (23.7374, 19.652) -> (23.5319, 19.2591)
  line L434 (23.5319, 19.2591) -> (23.3144, 18.8796)
  line L435 (23.3144, 18.8796) -> (23.0841, 18.5147)
  line L436 (23.0841, 18.5147) -> (22.84, 18.1661)
  line L437 (22.84, 18.1661) -> (22.7122, 17.9986)
  line L438 (22.7122, 17.9986) -> (22.6468, 17.9169)
  line L439 (22.6468, 17.9169) -> (22.5802, 17.8365)
  line L440 (22.5802, 17.8365) -> (23.0729, 17.1944)
  line L441 (23.0729, 17.1944) -> (23.1678, 17.2379)
  line L442 (23.1678, 17.2379) -> (23.2637, 17.2799)
  line L443 (23.2637, 17.2799) -> (23.4585, 17.36)
  line L444 (23.4585, 17.36) -> (23.8584, 17.5056)
  line L445 (23.8584, 17.5056) -> (24.2705, 17.6336)
  line L446 (24.2705, 17.6336) -> (24.6934, 17.7455)
  line L447 (24.6934, 17.7455) -> (25.1261, 17.8422)
  line L448 (25.1261, 17.8422) -> (25.5677, 17.9245)
  line L449 (25.5677, 17.9245) -> (25.8966, 17.446)
  line L450 (25.8966, 17.446) -> (25.6615, 17.0631)
  line L451 (25.6615, 17.0631) -> (25.4161, 16.6939)
  line L452 (25.4161, 16.6939) -> (25.1601, 16.3392)
  line L453 (25.1601, 16.3392) -> (24.8929, 16.0003)
  line L454 (24.8929, 16.0003) -> (24.6137, 15.6791)
  line L455 (24.6137, 15.6791) -> (24.4692, 15.526)
  line L456 (24.4692, 15.526) -> (24.3955, 15.4515)
  line L457 (24.3955, 15.4515) -> (24.3209, 15.3785)
  line L458 (24.3209, 15.3785) -> (24.7438, 14.6884)
  line L459 (24.7438, 14.6884) -> (24.8427, 14.7218)
  line L460 (24.8427, 14.7218) -> (24.9425, 14.7536)
  line L461 (24.9425, 14.7536) -> (25.1446, 14.8128)
  line L462 (25.1446, 14.8128) -> (25.5575, 14.9158)
  line L463 (25.5575, 14.9158) -> (25.9808, 15)
  line L464 (25.9808, 15) -> (26.413, 15.0671)
  line L465 (26.413, 15.0671) -> (26.8534, 15.1181)
  line L466 (26.8534, 15.1181) -> (27.3013, 15.1537)
  line L467 (27.3013, 15.1537) -> (27.5783, 14.6435)
  line L468 (27.5783, 14.6435) -> (27.3045, 14.2873)
  line L469 (27.3045, 14.2873) -> (27.0219, 13.9457)
  line L470 (27.0219, 13.9457) -> (26.7302, 13.6197)
  line L471 (26.7302, 13.6197) -> (26.4291, 13.3107)
  line L472 (26.4291, 13.3107) -> (26.1178, 13.0204)
  line L473 (26.1178, 13.0204) -> (25.958, 12.8832)
  line L474 (25.958, 12.8832) -> (25.877, 12.8168)
  line L475 (25.877, 12.8168) -> (25.7952, 12.752)
  line L476 (25.7952, 12.752) -> (26.1436, 12.0215)
  line L477 (26.1436, 12.0215) -> (26.2455, 12.0443)
  line L478 (26.2455, 12.0443) -> (26.348, 12.0655)
  line L479 (26.348, 12.0655) -> (26.5552, 12.1033)
  line L480 (26.5552, 12.1033) -> (26.9767, 12.1626)
  line L481 (26.9767, 12.1626) -> (27.4064, 12.2021)
  line L482 (27.4064, 12.2021) -> (27.8433, 12.2236)
  line L483 (27.8433, 12.2236) -> (28.2866, 12.2283)
  line L484 (28.2866, 12.2283) -> (28.7357, 12.2169)
  line L485 (28.7357, 12.2169) -> (28.9579, 11.6805)
  line L486 (28.9579, 11.6805) -> (28.6484, 11.3549)
  line L487 (28.6484, 11.3549) -> (28.3316, 11.0447)
  line L488 (28.3316, 11.0447) -> (28.0074, 10.751)
  line L489 (28.0074, 10.751) -> (27.6756, 10.4751)
  line L490 (27.6756, 10.4751) -> (27.3357, 10.219)
  line L491 (27.3357, 10.219) -> (27.1625, 10.0993)
  line L492 (27.1625, 10.0993) -> (27.075, 10.0417)
  line L493 (27.075, 10.0417) -> (26.9868, 9.9858)
  line L494 (26.9868, 9.9858) -> (27.257, 9.2229)
  line L495 (27.257, 9.2229) -> (27.3607, 9.235)
  line L496 (27.3607, 9.235) -> (27.4649, 9.2453)
  line L497 (27.4649, 9.2453) -> (27.6749, 9.2613)
  line L498 (27.6749, 9.2613) -> (28.1002, 9.2761)
  line L499 (28.1002, 9.2761) -> (28.5317, 9.2705)
  line L500 (28.5317, 9.2705) -> (28.9685, 9.2463)
  line L501 (28.9685, 9.2463) -> (29.4098, 9.2046)
  line L502 (29.4098, 9.2046) -> (29.8553, 9.1463)
  line L503 (29.8553, 9.1463) -> (30.0202, 8.5896)
  line L504 (30.0202, 8.5896) -> (29.6783, 8.2981)
  line L505 (29.6783, 8.2981) -> (29.3309, 8.0228)
  line L506 (29.3309, 8.0228) -> (28.9778, 7.7646)
  line L507 (28.9778, 7.7646) -> (28.619, 7.5249)
  line L508 (28.619, 7.5249) -> (28.2542, 7.3057)
  line L509 (28.2542, 7.3057) -> (28.0694, 7.2047)
  line L510 (28.0694, 7.2047) -> (27.9763, 7.1566)
  line L511 (27.9763, 7.1566) -> (27.8828, 7.1102)
  line L512 (27.8828, 7.1102) -> (28.0717, 6.3233)
  line L513 (28.0717, 6.3233) -> (28.1761, 6.3244)
  line L514 (28.1761, 6.3244) -> (28.2808, 6.3238)
  line L515 (28.2808, 6.3238) -> (28.4913, 6.3177)
  line L516 (28.4913, 6.3177) -> (28.9159, 6.288)
  line L517 (28.9159, 6.288) -> (29.3444, 6.2374)
  line L518 (29.3444, 6.2374) -> (29.7763, 6.1676)
  line L519 (29.7763, 6.1676) -> (30.2109, 6.08)
  line L520 (30.2109, 6.08) -> (30.6478, 5.9755)
  line L521 (30.6478, 5.9755) -> (30.7536, 5.4046)
  line L522 (30.7536, 5.4046) -> (30.3832, 5.1505)
  line L523 (30.3832, 5.1505) -> (30.0088, 4.9129)
  line L524 (30.0088, 4.9129) -> (29.6306, 4.693)
  line L525 (29.6306, 4.693) -> (29.2487, 4.4922)
  line L526 (29.2487, 4.4922) -> (28.863, 4.3123)
  line L527 (28.863, 4.3123) -> (28.6687, 4.2312)
  line L528 (28.6687, 4.2312) -> (28.5711, 4.1931)
  line L529 (28.5711, 4.1931) -> (28.4733, 4.1567)
  line L530 (28.4733, 4.1567) -> (28.5789, 3.3543)
  line L531 (28.5789, 3.3543) -> (28.6828, 3.3446)
  line L532 (28.6828, 3.3446) -> (28.7869, 3.333)
  line L533 (28.7869, 3.333) -> (28.9957, 3.305)
  line L534 (28.9957, 3.305) -> (29.4148, 3.231)
  line L535 (29.4148, 3.231) -> (29.8357, 3.1359)
  line L536 (29.8357, 3.1359) -> (30.2578, 3.0213)
  line L537 (30.2578, 3.0213) -> (30.6809, 2.8888)
  line L538 (30.6809, 2.8888) -> (31.1045, 2.7392)
  line L539 (31.1045, 2.7392) -> (31.1501, 2.1604)
  line L540 (31.1501, 2.1604) -> (30.7551, 1.9463)
  line L541 (30.7551, 1.9463) -> (30.3579, 1.7492)
  line L542 (30.3579, 1.7492) -> (29.9589, 1.5701)
  line L543 (29.9589, 1.5701) -> (29.5581, 1.4102)
  line L544 (29.5581, 1.4102) -> (29.1557, 1.2717)
  line L545 (29.1557, 1.2717) -> (28.9539, 1.2113)
  line L546 (28.9539, 1.2113) -> (28.8529, 1.1836)
  line L547 (28.8529, 1.1836) -> (28.7518, 1.1577)
  line L548 (28.7518, 1.1577) -> (28.773, 0.3487)
  line L549 (28.773, 0.3487) -> (28.8753, 0.3281)
  line L550 (28.8753, 0.3281) -> (28.9776, 0.3057)
  line L551 (28.9776, 0.3057) -> (29.1823, 0.256)
  line L552 (29.1823, 0.256) -> (29.5914, 0.1387)
  line L553 (29.5914, 0.1387) -> (30, 0)
  line L554 (30, 0) -> (30.4079, -0.158)
  line L555 (30.4079, -0.158) -> (30.8148, -0.3341)
  line L556 (30.8148, -0.3341) -> (31.2205, -0.5272)
  line L557 (31.2205, -0.5272) -> (31.2053, -1.1075)
  line L558 (31.2053, -1.1075) -> (30.7901, -1.2791)
  line L559 (30.7901, -1.2791) -> (30.3745, -1.4336)
  line L560 (30.3745, -1.4336) -> (29.9589, -1.5701)
  line L561 (29.9589, -1.5701) -> (29.5436, -1.6872)
  line L562 (29.5436, -1.6872) -> (29.1289, -1.7829)
  line L563 (29.1289, -1.7829) -> (28.9219, -1.8218)
  line L564 (28.9219, -1.8218) -> (28.8186, -1.8388)
  line L565 (28.8186, -1.8388) -> (28.7153, -1.854)
  line L566 (28.7153, -1.854) -> (28.6518, -2.6609)
  line L567 (28.6518, -2.6609) -> (28.7514, -2.692)
  line L568 (28.7514, -2.692) -> (28.8508, -2.725)
  line L569 (28.8508, -2.725) -> (29.0492, -2.7958)
  line L570 (29.0492, -2.7958) -> (29.4438, -2.9552)
  line L571 (29.4438, -2.9552) -> (29.8357, -3.1359)
  line L572 (29.8357, -3.1359) -> (30.2248, -3.3357)
  line L573 (30.2248, -3.3357) -> (30.6111, -3.5533)
  line L574 (30.6111, -3.5533) -> (30.9943, -3.7877)
  line L575 (30.9943, -3.7877) -> (30.9185, -4.3633)
  line L576 (30.9185, -4.3633) -> (30.4877, -4.4905)
  line L577 (30.4877, -4.4905) -> (30.0582, -4.6008)
  line L578 (30.0582, -4.6008) -> (29.6307, -4.693)
  line L579 (29.6307, -4.693) -> (29.2054, -4.7661)
  line L580 (29.2054, -4.7661) -> (28.7829, -4.8179)
  line L581 (28.7829, -4.8179) -> (28.5731, -4.835)
  line L582 (28.5731, -4.835) -> (28.4685, -4.8411)
  line L583 (28.4685, -4.8411) -> (28.3642, -4.8455)
  line L584 (28.3642, -4.8455) -> (28.2167, -5.6412)
  line L585 (28.2167, -5.6412) -> (28.3125, -5.6826)
  line L586 (28.3125, -5.6826) -> (28.408, -5.7258)
  line L587 (28.408, -5.7258) -> (28.5978, -5.8169)
  line L588 (28.5978, -5.8169) -> (28.9736, -6.0168)
  line L589 (28.9736, -6.0168) -> (29.3444, -6.2374)
  line L590 (29.3444, -6.2374) -> (29.7106, -6.4767)
  line L591 (29.7106, -6.4767) -> (30.072, -6.7335)
  line L592 (30.072, -6.7335) -> (30.4286, -7.0067)
  line L593 (30.4286, -7.0067) -> (30.2931, -7.5713)
  line L594 (30.2931, -7.5713) -> (29.8513, -7.6528)
  line L595 (29.8513, -7.6528) -> (29.4127, -7.7175)
  line L596 (29.4127, -7.7175) -> (28.9778, -7.7646)
  line L597 (28.9778, -7.7646) -> (28.5472, -7.7927)
  line L598 (28.5472, -7.7927) -> (28.1217, -7.8002)
  line L599 (28.1217, -7.8002) -> (27.9111, -7.7952)
  line L600 (27.9111, -7.7952) -> (27.8065, -7.7904)
  line L601 (27.8065, -7.7904) -> (27.7023, -7.7838)
  line L602 (27.7023, -7.7838) -> (27.4725, -8.5597)
  line L603 (27.4725, -8.5597) -> (27.5634, -8.611)
  line L604 (27.5634, -8.611) -> (27.6538, -8.6638)
  line L605 (27.6538, -8.6638) -> (27.8331, -8.7744)
  line L606 (27.8331, -8.7744) -> (28.1859, -9.0124)
  line L607 (28.1859, -9.0124) -> (28.5317, -9.2705)
  line L608 (28.5317, -9.2705) -> (28.8708, -9.5468)
  line L609 (28.8708, -9.5468) -> (29.2034, -9.84)
  line L610 (29.2034, -9.84) -> (29.5295, -10.149)
  line L611 (29.5295, -10.149) -> (29.3357, -10.6963)
  line L612 (29.3357, -10.6963) -> (28.8878, -10.7312)
  line L613 (28.8878, -10.7312) -> (28.4448, -10.7497)
  line L614 (28.4448, -10.7497) -> (28.0074, -10.751)
  line L615 (28.0074, -10.751) -> (27.5762, -10.7341)
  line L616 (27.5762, -10.7341) -> (27.1523, -10.697)
  line L617 (27.1523, -10.697) -> (26.9434, -10.67)
  line L618 (26.9434, -10.67) -> (26.8398, -10.6543)
  line L619 (26.8398, -10.6543) -> (26.7369, -10.6368)
  line L620 (26.7369, -10.6368) -> (26.4272, -11.3845)
  line L621 (26.4272, -11.3845) -> (26.5123, -11.4449)
  line L622 (26.5123, -11.4449) -> (26.5967, -11.507)
  line L623 (26.5967, -11.507) -> (26.7635, -11.6357)
  line L624 (26.7635, -11.6357) -> (27.0895, -11.9092)
  line L625 (27.0895, -11.9092) -> (27.4064, -12.2021)
  line L626 (27.4064, -12.2021) -> (27.7147, -12.5124)
  line L627 (27.7147, -12.5124) -> (28.0148, -12.8387)
  line L628 (28.0148, -12.8387) -> (28.3069, -13.1801)
  line L629 (28.3069, -13.1801) -> (28.057, -13.7041)
  line L630 (28.057, -13.7041) -> (27.6078, -13.692)
  line L631 (27.6078, -13.692) -> (27.1654, -13.6641)
  line L632 (27.1654, -13.6641) -> (26.7302, -13.6197)
  line L633 (26.7302, -13.6197) -> (26.3032, -13.5578)
  line L634 (26.3032, -13.5578) -> (25.8854, -13.4766)
  line L635 (25.8854, -13.4766) -> (25.6805, -13.4279)
  line L636 (25.6805, -13.4279) -> (25.5791, -13.4014)
  line L637 (25.5791, -13.4014) -> (25.4786, -13.3733)
  line L638 (25.4786, -13.3733) -> (25.0925, -14.0845)
  line L639 (25.0925, -14.0845) -> (25.1708, -14.1535)
  line L640 (25.1708, -14.1535) -> (25.2482, -14.2241)
  line L641 (25.2482, -14.2241) -> (25.4006, -14.3695)
  line L642 (25.4006, -14.3695) -> (25.6962, -14.6756)
  line L643 (25.6962, -14.6756) -> (25.9808, -15)
  line L644 (25.9808, -15) -> (26.255, -15.3408)
  line L645 (26.255, -15.3408) -> (26.5194, -15.6967)
  line L646 (26.5194, -15.6967) -> (26.7741, -16.0668)
  line L647 (26.7741, -16.0668) -> (26.4708, -16.5618)
  line L648 (26.4708, -16.5618) -> (26.0254, -16.5028)
  line L649 (26.0254, -16.5028) -> (25.5883, -16.4288)
  line L650 (25.5883, -16.4288) -> (25.1601, -16.3392)
  line L651 (25.1601, -16.3392) -> (24.7419, -16.2329)
  line L652 (24.7419, -16.2329) -> (24.3349, -16.1085)
  line L653 (24.3349, -16.1085) -> (24.1362, -16.0387)
  line L654 (24.1362, -16.0387) -> (24.0382, -16.0018)
  line L655 (24.0382, -16.0018) -> (23.9412, -15.9633)
  line L656 (23.9412, -15.9633) -> (23.4828, -16.6303)
  line L657 (23.4828, -16.6303) -> (23.5534, -16.7071)
  line L658 (23.5534, -16.7071) -> (23.6231, -16.7853)
  line L659 (23.6231, -16.7853) -> (23.7594, -16.9458)
  line L660 (23.7594, -16.9458) -> (24.0214, -17.2812)
  line L661 (24.0214, -17.2812) -> (24.2705, -17.6336)
  line L662 (24.2705, -17.6336) -> (24.5076, -18.0012)
  line L663 (24.5076, -18.0012) -> (24.7333, -18.3828)
  line L664 (24.7333, -18.3828) -> (24.948, -18.7774)
  line L665 (24.948, -18.7774) -> (24.5946, -19.238)
  line L666 (24.5946, -19.238) -> (24.1578, -19.1328)
  line L667 (24.1578, -19.1328) -> (23.7308, -19.0135)
  line L668 (23.7308, -19.0135) -> (23.3144, -18.8796)
  line L669 (23.3144, -18.8796) -> (22.9095, -18.7302)
  line L670 (22.9095, -18.7302) -> (22.5178, -18.5639)
  line L671 (22.5178, -18.5639) -> (22.3275, -18.4738)
  line L672 (22.3275, -18.4738) -> (22.2339, -18.4268)
  line L673 (22.2339, -18.4268) -> (22.1414, -18.3784)
  line L674 (22.1414, -18.3784) -> (21.6158, -18.9938)
  line L675 (21.6158, -18.9938) -> (21.6781, -19.0775)
  line L676 (21.6781, -19.0775) -> (21.7391, -19.1627)
  line L677 (21.7391, -19.1627) -> (21.8579, -19.3365)
  line L678 (21.8579, -19.3365) -> (22.0835, -19.6974)
  line L679 (22.0835, -19.6974) -> (22.2943, -20.0739)
  line L680 (22.2943, -20.0739) -> (22.4917, -20.4643)
  line L681 (22.4917, -20.4643) -> (22.6763, -20.8674)
  line L682 (22.6763, -20.8674) -> (22.8486, -21.2823)
  line L683 (22.8486, -21.2823) -> (22.4489, -21.7034)
  line L684 (22.4489, -21.7034) -> (22.0256, -21.5531)
  line L685 (22.0256, -21.5531) -> (21.6134, -21.3899)
  line L686 (21.6134, -21.3899) -> (21.2132, -21.2132)
  line L687 (21.2132, -21.2132) -> (20.8262, -21.0223)
  line L688 (20.8262, -21.0223) -> (20.454, -20.816)
  line L689 (20.454, -20.816) -> (20.2741, -20.7064)
  line L690 (20.2741, -20.7064) -> (20.1859, -20.6499)
  line L691 (20.1859, -20.6499) -> (20.099, -20.5921)
  line L692 (20.099, -20.5921) -> (19.512, -21.1492)
  line L693 (19.512, -21.1492) -> (19.5652, -21.239)
  line L694 (19.5652, -21.239) -> (19.617, -21.33)
  line L695 (19.617, -21.33) -> (19.717, -21.5154)
  line L696 (19.717, -21.5154) -> (19.9035, -21.8979)
  line L697 (19.9035, -21.8979) -> (20.0739, -22.2943)
  line L698 (20.0739, -22.2943) -> (20.2294, -22.7032)
  line L699 (20.2294, -22.7032) -> (20.3709, -23.1234)
  line L700 (20.3709, -23.1234) -> (20.4988, -23.5541)
  line L701 (20.4988, -23.5541) -> (20.0573, -23.9311)
  line L702 (20.0573, -23.9311) -> (19.652, -23.7374)
  line L703 (19.652, -23.7374) -> (19.2591, -23.5319)
  line L704 (19.2591, -23.5319) -> (18.8796, -23.3144)
  line L705 (18.8796, -23.3144) -> (18.5147, -23.0841)
  line L706 (18.5147, -23.0841) -> (18.1661, -22.84)
  line L707 (18.1661, -22.84) -> (17.9986, -22.7122)
  line L708 (17.9986, -22.7122) -> (17.9169, -22.6468)
  line L709 (17.9169, -22.6468) -> (17.8365, -22.5802)
  line L710 (17.8365, -22.5802) -> (17.1944, -23.0729)
  line L711 (17.1944, -23.0729) -> (17.2379, -23.1678)
  line L712 (17.2379, -23.1678) -> (17.2799, -23.2637)
  line L713 (17.2799, -23.2637) -> (17.36, -23.4585)
  line L714 (17.36, -23.4585) -> (17.5056, -23.8584)
  line L715 (17.5056, -23.8584) -> (17.6336, -24.2705)
  line L716 (17.6336, -24.2705) -> (17.7455, -24.6934)
  line L717 (17.7455, -24.6934) -> (17.8422, -25.1261)
  line L718 (17.8422, -25.1261) -> (17.9245, -25.5677)
  line L719 (17.9245, -25.5677) -> (17.446, -25.8966)
  line L720 (17.446, -25.8966) -> (17.0631, -25.6615)
  line L721 (17.0631, -25.6615) -> (16.6939, -25.4161)
  line L722 (16.6939, -25.4161) -> (16.3392, -25.1601)
  line L723 (16.3392, -25.1601) -> (16.0003, -24.8929)
  line L724 (16.0003, -24.8929) -> (15.6791, -24.6137)
  line L725 (15.6791, -24.6137) -> (15.526, -24.4692)
  line L726 (15.526, -24.4692) -> (15.4515, -24.3955)
  line L727 (15.4515, -24.3955) -> (15.3785, -24.3209)
  line L728 (15.3785, -24.3209) -> (14.6884, -24.7438)
  line L729 (14.6884, -24.7438) -> (14.7218, -24.8427)
  line L730 (14.7218, -24.8427) -> (14.7536, -24.9425)
  line L731 (14.7536, -24.9425) -> (14.8128, -25.1446)
  line L732 (14.8128, -25.1446) -> (14.9158, -25.5576)
  line L733 (14.9158, -25.5576) -> (15, -25.9808)
  line L734 (15, -25.9808) -> (15.0671, -26.413)
  line L735 (15.0671, -26.413) -> (15.1181, -26.8534)
  line L736 (15.1181, -26.8534) -> (15.1537, -27.3013)
  line L737 (15.1537, -27.3013) -> (14.6435, -27.5783)
  line L738 (14.6435, -27.5783) -> (14.2873, -27.3045)
  line L739 (14.2873, -27.3045) -> (13.9457, -27.0219)
  line L740 (13.9457, -27.0219) -> (13.6197, -26.7302)
  line L741 (13.6197, -26.7302) -> (13.3107, -26.4291)
  line L742 (13.3107, -26.4291) -> (13.0204, -26.1178)
  line L743 (13.0204, -26.1178) -> (12.8832, -25.958)
  line L744 (12.8832, -25.958) -> (12.8168, -25.877)
  line L745 (12.8168, -25.877) -> (12.752, -25.7952)
  line L746 (12.752, -25.7952) -> (12.0215, -26.1436)
  line L747 (12.0215, -26.1436) -> (12.0443, -26.2455)
  line L748 (12.0443, -26.2455) -> (12.0655, -26.3481)
  line L749 (12.0655, -26.3481) -> (12.1033, -26.5552)
  line L750 (12.1033, -26.5552) -> (12.1626, -26.9767)
  line L751 (12.1626, -26.9767) -> (12.2021, -27.4064)
  line L752 (12.2021, -27.4064) -> (12.2236, -27.8433)
  line L753 (12.2236, -27.8433) -> (12.2283, -28.2866)
  line L754 (12.2283, -28.2866) -> (12.2169, -28.7357)
  line L755 (12.2169, -28.7357) -> (11.6805, -28.9579)
  line L756 (11.6805, -28.9579) -> (11.3549, -28.6484)
  line L757 (11.3549, -28.6484) -> (11.0447, -28.3316)
  line L758 (11.0447, -28.3316) -> (10.751, -28.0074)
  line L759 (10.751, -28.0074) -> (10.4751, -27.6756)
  line L760 (10.4751, -27.6756) -> (10.219, -27.3357)
  line L761 (10.219, -27.3357) -> (10.0993, -27.1625)
  line L762 (10.0993, -27.1625) -> (10.0417, -27.075)
  line L763 (10.0417, -27.075) -> (9.9858, -26.9868)
  line L764 (9.9858, -26.9868) -> (9.2229, -27.257)
  line L765 (9.2229, -27.257) -> (9.235, -27.3607)
  line L766 (9.235, -27.3607) -> (9.2453, -27.4649)
  line L767 (9.2453, -27.4649) -> (9.2613, -27.6749)